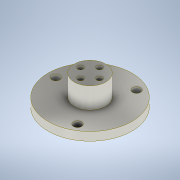
# Autodesk Inventor part: Planet_Gear_Output
Saved by Autodesk Inventor 2022.3 (Build 263350000, 350)
## iProperties
Created: 2022-04-22
Part Number: Planet_Gear_Output
Material: Generic
Document SubType Name: Modeling
Designer: Mlees
Density: 1 g/cm^3
Appearance: Silver
Mass: 4.19966 g
Surface Area: 23.4388 cm^2
Volume: 4.19966 cm^3
Author: Mlees
Autodesk Inventor part; units mm, degrees
ref_plane "YZ Plane" through (0, 0, 0) normal (1, 0, 0) x (0, 1, 0)
ref_plane "XZ Plane" through (0, 0, 0) normal (0, 1, 0) x (-1, 0, 0)
ref_plane "XY Plane" through (0, 0, 0) normal (0, 0, 1) x (1, 0, 0)
sketch "Sketch1" plane through (0, 0, 0) normal (0, 1, 0) x (-1, 0, 0)
  circle A0 centre (16.272, 0) radius 1.95
  line L0 (14.741, 3.5) -> (19.6914, 3.5)
  line L1 (14.741, -3.5) -> (19.6914, -3.5)
  line L2 (14.741, 3.5) -> (12, 3.5)
  line L3 (14.741, -3.5) -> (12, -3.5)
  line L4 (-2.9689, 12.1423) -> (-6.8146, 18.8032)
  line L5 (-12.8768, 15.3032) -> (-9.0311, 8.6423)
  line L6 (12, -3.5) -> (19.6914, -3.5)
  line L7 (12, 3.5) -> (19.6914, 3.5)
  line L8 (-2.9689, -12.1423) -> (-6.8146, -18.8032)
  line L9 (-9.0311, -8.6423) -> (-12.8768, -15.3032)
  arc A1 (-6.8146, 18.8032) -> (-12.8768, 15.3032) centre (0, 0) ccw
  arc A2 (-12.8768, -15.3032) -> (-6.8146, -18.8032) centre (0, 0) ccw
  arc A3 (19.6914, -3.5) -> (19.6914, 3.5) centre (0, 0) ccw
  arc A4 (-9.0311, 8.6423) -> (-9.0311, -8.6423) centre (0, 0) ccw
  arc A5 (-2.9689, -12.1423) -> (12, -3.5) centre (0, 0) ccw
  arc A6 (12, 3.5) -> (-2.9689, 12.1423) centre (0, 0) ccw
  line L10 (0, 0) -> (16.272, 0)
  circle A7 centre (-8.136, 14.092) radius 1.95
  circle A8 centre (-8.136, -14.092) radius 1.95
  dimension "d6" = 3.9
  dimension "d20" = 16.272
  dimension "d23" = 360
  constraints: 22 end point, 12 point on circle, 9 centre point, 3 horizontal, 1 coincident, 1 collinear, 1 parallel, 7 other
  measures "d6" diameter of A0
  measures "d20" distance of L10.start L10.end
extrude "Extrusion1" add sketch "Sketch1" along normal blind 4
sketch "Sketch2" plane through (0, 4, 0) normal (0, 1, 0) x (1, 0, 0)
  circle A0 centre (0, 0) radius 7.5
  constraints: 1 centre point, 1 coincident
extrude "Extrusion2" add sketch "Sketch2" along normal blind 6
sketch "Sketch3" plane through (0, 10, 0) normal (0, 1, 0) x (1, 0, 0)
  circle A0 centre (-4.5, 0) radius 1.35
  circle A1 centre (0, -4.5) radius 1.35
  circle A2 centre (4.5, 0) radius 1.35
  circle A3 centre (0, 4.5) radius 1.35
  point P0 (0, 0)
  point P1 (0, 0)
  dimension "d26" = 2.7
  dimension "d30" = 360
  constraints: 4 centre point, 1 coincident, 9 other
  measures "d26" diameter of A0
extrude "Extrusion3" cut sketch "Sketch3" against normal through all
sketch "Sketch4" plane through (0, 0, 0) normal (0, -1, 0) x (1, 0, 0)
  circle A0 centre (-4.5, 0) radius 1.35 projected
  circle A1 centre (-4.5, 0) radius 2
  circle A2 centre (0, -4.5) radius 2
  circle A3 centre (4.5, 0) radius 2
  circle A4 centre (0, 4.5) radius 2
  point P0 (0, 0)
  point P1 (0, 0)
  dimension "d34" = 4
  dimension "d37" = 360
  constraints: 4 centre point, 2 coincident, 9 other
  measures "d34" diameter of A1
extrude "Extrusion4" cut sketch "Sketch4" against normal blind 3
sketch "Sketch5" plane through (0, 0, 0) normal (0, -1, 0) x (1, 0, 0)
  arc A0 (12.8768, 15.3032) -> (6.8146, 18.8032) centre (0, 0) ccw projected
  arc A1 (-19.6914, 3.5) -> (-19.6914, -3.5) centre (0, 0) ccw projected
  line L0 (-19.6914, 3.5) -> (-12, 3.5) projected
  line L1 (-19.6914, 3.5) -> (-12, 3.5)
  line L2 (-12, -3.5) -> (-19.6914, -3.5) projected
  line L3 (-19.6914, -3.5) -> (-12, -3.5)
  line L4 (6.8146, -18.8032) -> (2.9689, -12.1423) projected
  line L5 (6.8146, -18.8032) -> (2.9689, -12.1423)
  line L6 (9.0311, -8.6423) -> (12.8768, -15.3032) projected
  line L7 (12.8768, -15.3032) -> (9.0311, -8.6423)
  line L8 (12.8768, 15.3032) -> (9.0311, 8.6423) projected
  arc A2 (9.0311, -8.6423) -> (9.0311, 8.6423) centre (0, 0) ccw projected
  line L9 (12.8768, 15.3032) -> (9.0311, 8.6423)
  line L10 (2.9689, 12.1423) -> (6.8146, 18.8032) projected
  line L11 (6.8146, 18.8032) -> (2.9689, 12.1423)
  arc A3 (2.9689, 12.1423) -> (-12, 3.5) centre (0, 0) ccw projected
  arc A4 (2.9689, 12.1423) -> (-12, 3.5) centre (0, 0) ccw
  arc A5 (6.8146, 18.8032) -> (-19.6914, 3.5) centre (0, 0) ccw
  arc A6 (-19.6914, -3.5) -> (6.8146, -18.8032) centre (0, 0) ccw
  arc A7 (12.8768, -15.3032) -> (12.8768, 15.3032) centre (0, 0) ccw
  arc A8 (-12, -3.5) -> (2.9689, -12.1423) centre (0, 0) ccw
  arc A9 (9.0311, -8.6423) -> (9.0311, 8.6423) centre (0, 0) ccw
  constraints: 13 end point, 12 point on circle, 6 centre point, 3 collinear, 2 coincident, 2 horizontal
extrude "Extrusion5" add sketch "Sketch5" against normal up to surface (4 mm away)
fillet "Fillet1" radius 1 3 edges at (10.086, 0, 14.092) (-14.322, 0, 0) (10.086, 0, -14.092)
sketch "Sketch6" plane through (0, 10, 0) normal (0, 1, 0) x (1, 0, 0)
  circle A0 centre (0, 0) radius 7.5
  circle A1 centre (-4.5, 0) radius 1.35 projected
  circle A2 centre (-4.5, 0) radius 1.35
  circle A3 centre (0, 4.5) radius 1.35 projected
  circle A4 centre (0, 4.5) radius 1.35
  circle A5 centre (4.5, 0) radius 1.35 projected
  circle A6 centre (4.5, 0) radius 1.35
  circle A7 centre (0, -4.5) radius 1.35 projected
  circle A8 centre (0, -4.5) radius 1.35
  constraints: 5 centre point, 5 coincident
extrude "Extrusion6" add sketch "Sketch6" along normal blind 4
body "Solid1"
